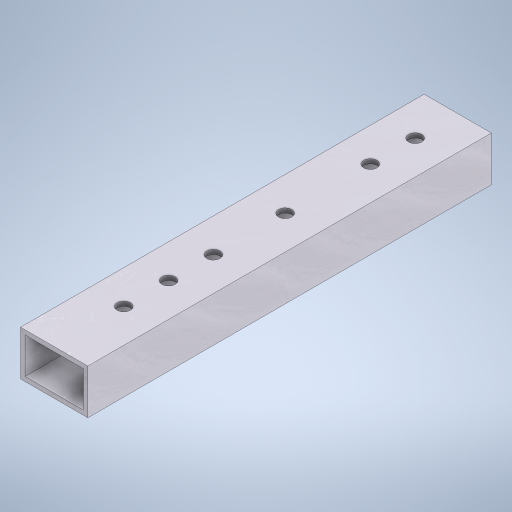
# Autodesk Inventor part: profile4
Saved by Autodesk Inventor 2023 (Build 270158000, 158)
## iProperties
Created: 2024-02-07
Part Number: profile4
Material: Aluminum 6061, Welded
Document SubType Name: Modeling
Designer: victo
Density: 2.7 g/cm^3
Appearance: Weld - Aluminum
Author: victo
Autodesk Inventor part; units mm, degrees
ref_plane "YZ Plane" through (0, 0, 0) normal (1, 0, 0) x (0, 1, 0)
ref_plane "XZ Plane" through (0, 0, 0) normal (0, 1, 0) x (-1, 0, 0)
ref_plane "XY Plane" through (0, 0, 0) normal (0, 0, 1) x (1, 0, 0)
sketch "Sketch1" plane through (0, 0, 0) normal (0, 0, 1) x (1, 0, 0)
  line L0 (0, 0) -> (15, 0)
  line L1 (15, 0) -> (15, 10)
  line L2 (15, 10) -> (0, 10)
  line L3 (0, 10) -> (0, 0)
  line L4 (1, 9) -> (14, 9)
  line L5 (14, 9) -> (14, 1)
  line L6 (14, 1) -> (1, 1)
  line L7 (1, 1) -> (1, 9)
  dimension "d0" = 15
  dimension "d1" = 10
  dimension "d2" = 13
  dimension "d3" = 8
  dimension "d4" = 1
  dimension "d5" = 1
  constraints: 16 end point, 4 parallel, 2 horizontal, 2 perpendicular
  measures "d0" distance of L2.end L1.end
  measures "d1" distance of L1.end L0.end
  measures "d2" distance of L5.end L6.end
  measures "d3" distance of L4.end L5.end
  measures "d4" distance between parallel lines of L3 L7
  measures "d5" distance between parallel lines of L2 L4
extrude "Extrusion1" add sketch "Sketch1" along normal blind 90
sketch "Sketch2" plane through (0, 10, 0) normal (0, 1, 0) x (1, 0, 0)
  line L0 (15, 0) -> (0, 0) projected
  line L1 (0, 0) -> (0, -90) projected
  line L2 (15, -90) -> (0, -90) projected
  line L3 (15, 0) -> (15, -90) projected
  circle A0 centre (7.5, -9.5) radius 1.5
  circle A1 centre (7.5, -74.5) radius 1.5
  circle A2 centre (7.5, -19.5) radius 1.5
  circle A3 centre (7.5, -64.5) radius 1.5
  circle A4 centre (7.5, -54.5) radius 1.5
  circle A5 centre (7.5, -38.5) radius 1.5
  dimension "d8" = 3
  dimension "d9" = 3
  dimension "d10" = 7.5
  dimension "d11" = 7.5
  dimension "d12" = 9.5
  dimension "d13" = 15.5
  dimension "d24" = 3
  dimension "d25" = 3
  dimension "d26" = 3
  dimension "d27" = 3
  dimension "d28" = 7.5
  dimension "d29" = 7.5
  dimension "d30" = 7.5
  dimension "d31" = 7.5
  dimension "d32" = 10
  dimension "d33" = 10
  dimension "d34" = 10
  dimension "d35" = 16
  constraints: 6 centre point
  measures "d8" diameter of A0
  measures "d9" diameter of A1
  measures "d10" distance from line of L1 A0.centre
  measures "d11" distance from line of L1 A1.centre
  measures "d12" distance from line of L0 A0.centre
  measures "d13" distance from line of L2 A1.centre
  measures "d24" diameter of A2
  measures "d25" diameter of A3
  measures "d26" diameter of A4
  measures "d27" diameter of A5
  measures "d28" distance from line of L1 A3.centre
  measures "d29" distance from line of L1 A4.centre
  measures "d30" distance from line of L1 A5.centre
  measures "d31" distance from line of L1 A2.centre
  measures "d32" distance of A0.centre A2.centre
  measures "d33" distance of A1.centre A3.centre
  measures "d34" distance of A3.centre A4.centre
  measures "d35" distance of A4.centre A5.centre
extrude "Extrusion2" cut sketch "Sketch2" against normal up to surface (10 mm away) contours A0 | A1 | A2 | A3 | A4 | A5
sketch "Sketch3" plane through (15, 0, 0) normal (1, 0, 0) x (0, 0, -1)
  line L0 (0, 0) -> (0, 10) projected
  line L1 (0, 10) -> (-90, 10) projected
  line L2 (-90, 0) -> (-90, 10) projected
  line L3 (0, 0) -> (-90, 0) projected
  circle A0 centre (-9, 5) radius 1.5
  circle A1 centre (-85, 5) radius 1.5
  dimension "d16" = 3
  dimension "d17" = 5
  dimension "d18" = 9
  dimension "d21" = 3
  dimension "d22" = 5
  dimension "d23" = 5
  constraints: 2 centre point
  measures "d16" diameter of A0
  measures "d17" distance from line of L1 A0.centre
  measures "d18" distance from line of L0 A0.centre
  measures "d21" diameter of A1
  measures "d22" distance from line of L1 A1.centre
  measures "d23" distance from line of L2 A1.centre
extrude "Extrusion3" [suppressed]
body "Solid1"
